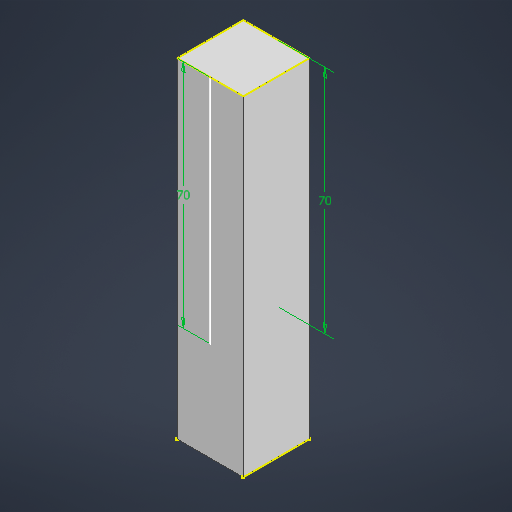
# Autodesk Inventor part: Main_Pole
Saved by Autodesk Inventor 2026.1 (Build 301233000, 233)
## iProperties
Created: 2025-09-01
Part Number: Main_Pole
Material: Generic
Document SubType Name: Modeling
Designer: junha
Density: 1 g/cm^3
Appearance: Default
Author: junha
Autodesk Inventor part; units mm, degrees
ref_plane "YZ Plane" through (0, 0, 0) normal (1, 0, 0) x (0, 1, 0)
ref_plane "XZ Plane" through (0, 0, 0) normal (0, 1, 0) x (-1, 0, 0)
ref_plane "XY Plane" through (0, 0, 0) normal (0, 0, 1) x (1, 0, 0)
sketch "Sketch1" plane through (0, 0, 0) normal (0, 1, 0) x (-1, 0, 0)
  line L0 (0, 0) -> (0, -20)
  line L1 (0, -20) -> (20, -20)
  line L2 (20, -20) -> (20, 0)
  line L3 (20, 0) -> (0, 0)
  dimension "d0" = 20
  dimension "d1" = 20
  constraints: 8 end point, 3 perpendicular, 1 vertical
  measures "d0" distance of L0.start L0.end
  measures "d1" distance of L0.end L1.end
extrude "Extrusion1" add sketch "Sketch1" along normal blind 90
sketch "Sketch2" plane through (0, 90, 0) normal (0, 1, 0) x (1, 0, 0)
  line L0 (-20, 20) -> (-20, 0) projected
  line L1 (-20, 20) -> (0, 20)
  line L2 (0, 20) -> (0, 0)
  line L3 (0, 0) -> (-20, 0)
  line L4 (-20, 0) -> (-20, 20)
  constraints: 8 end point, 2 parallel, 1 horizontal, 1 perpendicular
extrude "Extrusion2" add sketch "Sketch2" along normal blind 10
sketch "Sketch3" plane through (0, 0, 0) normal (1, 0, 0) x (0, 0, -1)
  line L0 (20, 0) -> (0, 0) projected
  line L1 (0, 100) -> (20, 100) projected
sketch "Sketch4" plane through (-20, 0, -20) normal (-1, 0, 0) x (0, 0, 1)
  line L0 (0, 100) -> (20, 100) projected
  point P0 (20, 0)
sketch "Sketch5" plane through (-20, 0, 0) normal (0, 0, 1) x (1, 0, 0)
  line L0 (0, 100) -> (20, 100) projected
  line L1 (10, 100) -> (10, 30)
  point P0 (20, 0)
  dimension "d9" = 70
  constraints: 2 end point, 1 midpoint, 1 vertical
  measures "d9" distance of L1.start L1.end
sketch "Sketch6" plane through (0, 0, -20) normal (0, 0, -1) x (-1, 0, 0)
  line L0 (20, 100) -> (0, 100) projected
  line L1 (10, 100) -> (10, 30)
  point P0 (0, 0)
  dimension "d10" = 70
  constraints: 2 end point, 1 midpoint, 1 vertical
  measures "d10" distance of L1.start L1.end
body "Solid1"
